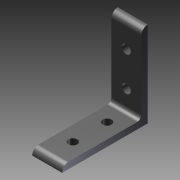
# Autodesk Inventor part: 4101
Saved by Autodesk Inventor 2011 SP1 (Build 150282100, 282)
## iProperties
Created: 2017-04-21
Part Number: 4101
Catalog Web Link: www.cadenas.de
Description: 4101-Joining Plates - 4 Hole 2.5 Inch Inside Corner Bracket
Vendor: 8020
Document SubType Name: Modeling
Designer: psAdmin
Manufacturer: 8020
Mass: 12.1629 g
Surface Area: 67.9978 cm^2
Volume: 12.1629 cm^3
Density: 1 g/cm^3
Category: PARTsolutions
Company: 8020
Title: 4101
Author: Cadenas PARTsolutions
Comments: Joining Plates - 4 Hole 2.5 Inch Inside Corner Bracket
PSOL_IDENT_0: {$CADENAS_DATA\23d-libs\8020\inch\joining_plates\4101.prj},139 {VTYP=3D},{NB=4101},{LINA=4101},{NN=4
PSOL_IDENT_1: 101},{DATE=22.08.2012},{GEOMDATE=07.12.2011 08:25:00},{VERSION=},{LINEID=10},{LINESUBID=-1},{WBVAR=}
PSOL_IDENT_2: {NB=4101},{LINA=4101},{KT=DUMMY},{PN=4101},{A=0.875},{B=0.750},{C=1.000},{D=2.500},{E=0.257},{W=.0
PSOL_IDENT_3: 75},{D1=0.188},{R=0.125}
NN: 4101
NT: Joining Plates - 4 Hole 2.5 Inch Inside Corner Bracket
NB: 4101
NBSYN: $PN.
LINA: 4101
PN: 4101
A: 0.875
B: 0.750
C: 1.000
D: 2.500
E: 0.257
W: .075
SUPPLIER: 8020
ARTICLENO: 4101
BOMINFO: 4101
CREATOR: CADENAS GmbH
Autodesk Inventor part; units mm, degrees
ref_plane "YZ Plane" through (0, 0, 0) normal (1, 0, 0) x (0, 1, 0)
ref_plane "XZ Plane" through (0, 0, 0) normal (0, 1, 0) x (-1, 0, 0)
ref_plane "XY Plane" through (0, 0, 0) normal (0, 0, 1) x (1, 0, 0)
sketch "Sketch_1" plane through (0, 0, 0) normal (1, 0, 0) x (0, 1, 0)
  line L0 (0, 63.5) -> (0, 0)
  line L1 (0, 0) -> (63.5, 0)
  arc A0 (63.5, 0) -> (58.7248, 4.7752) centre (58.7248, 0) ccw
  line L2 (58.7248, 4.7752) -> (7.9502, 4.7752)
  arc A1 (4.7752, 7.9502) -> (7.9502, 4.7752) centre (7.9502, 7.9502) ccw
  line L3 (4.7752, 7.9502) -> (4.7752, 58.7248)
  arc A2 (4.7752, 58.7248) -> (0, 63.5) centre (0, 58.7248) ccw
  constraints: 8 end point, 6 point on circle, 3 centre point
extrude "Extrusion1" add sketch "Sketch_1" along normal mid plane 22.225
sketch "Sketch2" plane through (11.1125, 0, 0) normal (0, 0, -1) x (-1, 0, 0)
  point P0 (11.1125, 19.05)
hole "Hole1" at (0, 19.05, 0) direction (0, 0, 1) diameter 6.5278 depth 4.7752
sketch "Sketch3" plane through (11.1125, 0, 0) normal (0, 0, -1) x (-1, 0, 0)
  point P0 (11.1125, 44.45)
hole "Hole2" at (0, 44.45, 0) direction (0, 0, 1) diameter 6.5278 depth 4.7752
sketch "Sketch4" plane through (-11.1125, 0, 63.5) normal (0, -1, 0) x (1, 0, 0)
  point P0 (11.1125, -44.45)
hole "Hole3" at (0, 0, 19.05) direction (0, 1, 0) diameter 6.5278 depth 4.7752
sketch "Sketch5" plane through (-11.1125, 0, 63.5) normal (0, -1, 0) x (1, 0, 0)
  point P0 (11.1125, -19.05)
hole "Hole4" at (0, 0, 44.45) direction (0, 1, 0) diameter 6.5278 depth 4.7752
body "Solid1"
